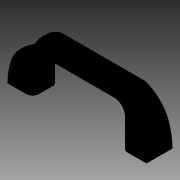
# Autodesk Inventor part: 2062
Saved by Autodesk Inventor 2014 SP2 (Build 180246200, 246)
## iProperties
Created: 2018-07-23
Part Number: 2062
Material: Generic
Catalog Web Link: www.cadenas.de
Description: 2060, 2061, 2062, 2880, 2881, 2882-Plastic Door Handles
Vendor: 8020
Document SubType Name: Modeling
Designer: psadmin
Manufacturer: 8020
Mass: 22.5234 g
Surface Area: 109.46 cm^2
Volume: 22.5234 cm^3
Density: 1 g/cm^3
Appearance: PSOLRGB-0-0-0
Category: PARTsolutions
Company: 8020
Title: 2062
Author: Cadenas PARTsolutions
Comments: Plastic Door Handles
PSOL_IDENT_0: {$CADENAS_DATA\23d-libs\8020\inch\panels_and_doors\2060.prj},182 {VTYP=3D},{NB=2062},{LINA=2062},{NN=
PSOL_IDENT_1: 2060, 2061, 2062, 2880, 2881, 2882},{DATE=16.03.2018 08:23:48},{GEOMDATE=03.01.2012 00:00:00},{VERSI
PSOL_IDENT_2: ON=},{LINEID=330},{WBVAR=COLOR},{WBNUMERIC=}  {NB=2062},{LINA=2062},{KT=DUMMY},{PN=2062},{SIZE=Small
PSOL_IDENT_3: },{MAT=High Strength Polycarbonate},{COLOR=Black},{A=4.409},{B=2.815},{C=1.417},{D=0.827},{E=3.681},
PSOL_IDENT_4: {F=1/4-20 SHCS (2)},{W=.055},{CC=6-10, 6-25},{COL=0.00,0.00,0.00,0.00}
NN: 2060, 2061, 2062, 2880, 2881, 2882
NT: Plastic Door Handles
NB: 2062
NBSYN: $PN.
LINA: 2062
PN: 2062
SIZE: Small
MAT: High Strength Polycarbonate
COLOR: Black
A: 4.409
B: 2.815
C: 1.417
D: 0.827
E: 3.681
F: 1/4-20 SHCS (2)
W: .055
CC: 6-10, 6-25
SUPPLIER: 8020
ARTICLENO: 2062
BOMINFO: 2062
CREATOR: CADENAS GmbH
Autodesk Inventor part; units mm, degrees
ref_plane "YZ Plane" through (0, 0, 0) normal (1, 0, 0) x (0, 1, 0)
ref_plane "XZ Plane" through (0, 0, 0) normal (0, 1, 0) x (-1, 0, 0)
ref_plane "XY Plane" through (0, 0, 0) normal (0, 0, 1) x (1, 0, 0)
sketch "Sketch_19" plane through (0, 0, 0) normal (0, 1, 0) x (-1, 0, 0)
  line L0 (20.2438, -10.5029) -> (20.2438, 10.5029)
  line L1 (20.2438, 10.5029) -> (5, 10.5029)
  arc A0 (5, 10.5029) -> (0, 5.5029) centre (5, 5.5029) ccw
  line L2 (0, 5.5029) -> (0, -5.5029)
  arc A1 (0, -5.5029) -> (5, -10.5029) centre (5, -5.5029) ccw
  line L3 (5, -10.5029) -> (20.2438, -10.5029)
  constraints: 8 end point, 4 point on circle, 2 centre point
extrude "Extrusion1" add sketch "Sketch_19" along normal blind 22.9918
sketch "Sketch_20" plane through (0, 22.9918, 0) normal (0, 1, 0) x (1, 0, 0)
  line L0 (7, 5.5029) -> (7, -5.5029)
  line L1 (-20.2438, 10.5029) -> (-20.2438, -10.5029)
  line L2 (-20.2438, -10.5029) -> (-5, -10.5029)
  arc A0 (-5, -10.5029) -> (0, -5.5029) centre (-5, -5.5029) ccw
  line L3 (0, -5.5029) -> (0, 5.5029)
  arc A1 (0, 5.5029) -> (-5, 10.5029) centre (-5, 5.5029) ccw
  line L4 (-5, 10.5029) -> (-20.2438, 10.5029)
  constraints: 10 end point, 4 point on circle, 2 centre point
revolve "Revolution1" add sketch "Sketch_20" angle 90 about axis through (7, 22.9918, -5.5029) along (0, 0, -1)
sketch "Sketch_21" plane through (7, 0, 0) normal (1, 0, 0) x (0, 0, -1)
  arc A0 (-10.5029, 34.9918) -> (-5.5029, 29.9918) centre (-5.5029, 34.9918) ccw
  line L0 (-5.5029, 29.9918) -> (5.5029, 29.9918)
  arc A1 (5.5029, 29.9918) -> (10.5029, 34.9918) centre (5.5029, 34.9918) ccw
  line L1 (10.5029, 34.9918) -> (10.5029, 50.2356)
  line L2 (10.5029, 50.2356) -> (-10.5029, 50.2356)
  line L3 (-10.5029, 50.2356) -> (-10.5029, 34.9918)
  constraints: 8 end point, 4 point on circle, 2 centre point
extrude "Extrusion2" add sketch "Sketch_21" along normal blind 57.501
sketch "Sketch_22" plane through (64.501, 0, 0) normal (1, 0, 0) x (0, 0, -1)
  line L0 (5.5029, 22.9918) -> (-5.5029, 22.9918)
  arc A0 (-10.5029, 34.9918) -> (-5.5029, 29.9918) centre (-5.5029, 34.9918) ccw
  line L1 (-5.5029, 29.9918) -> (5.5029, 29.9918)
  arc A1 (5.5029, 29.9918) -> (10.5029, 34.9918) centre (5.5029, 34.9918) ccw
  line L2 (10.5029, 34.9918) -> (10.5029, 50.2356)
  line L3 (10.5029, 50.2356) -> (-10.5029, 50.2356)
  line L4 (-10.5029, 50.2356) -> (-10.5029, 34.9918)
  constraints: 10 end point, 4 point on circle, 2 centre point
revolve "Revolution2" add sketch "Sketch_22" angle 90 about axis through (64.501, 22.9918, -5.5029) along (0, 0, -1)
sketch "Sketch_23" plane through (0, 0, 0) normal (0, 1, 0) x (-1, 0, 0)
  arc A0 (-71.501, 5.5029) -> (-76.501, 10.5029) centre (-76.501, 5.5029) ccw
  line L0 (-76.501, 10.5029) -> (-91.7448, 10.5029)
  line L1 (-91.7448, 10.5029) -> (-91.7448, -10.5029)
  line L2 (-91.7448, -10.5029) -> (-76.501, -10.5029)
  arc A1 (-76.501, -10.5029) -> (-71.501, -5.5029) centre (-76.501, -5.5029) ccw
  line L3 (-71.501, -5.5029) -> (-71.501, 5.5029)
  constraints: 8 end point, 4 point on circle, 2 centre point
extrude "Extrusion3" add sketch "Sketch_23" along normal blind 22.9918
sketch "Sketch_24" plane through (0, 0, 0) normal (0, 0, 1) x (1, 0, 0)
  line L0 (-32.9438, 71.9836) -> (-32.9438, 0)
  line L1 (-32.9438, 0) -> (-20.2438, 0)
  arc A0 (-18.4912, 13.0048) -> (-20.2438, 0) centre (34.459, -0.7516) ccw
  arc A1 (2.0066, 35.9918) -> (-18.4912, 13.0048) centre (10.8872, 7.4403) ccw
  line L2 (2.0066, 35.9918) -> (69.4944, 35.9918)
  arc A2 (89.9922, 13.0048) -> (69.4944, 35.9918) centre (60.6138, 7.4403) ccw
  arc A3 (91.7448, 0) -> (89.9922, 13.0048) centre (37.042, -0.7516) ccw
  line L3 (91.7448, 0) -> (104.4448, 0)
  line L4 (104.4448, 0) -> (104.4448, 71.9836)
  line L5 (104.4448, 71.9836) -> (-32.9438, 71.9836)
  constraints: 12 end point, 8 point on circle, 4 centre point
extrude "Extrusion4" cut sketch "Sketch_24" along normal mid plane 42.0116
sketch "Sketch_25" plane through (0, 0, 0) normal (0, 0, 1) x (1, 0, 0)
  line L0 (82.4992, 0) -> (82.4992, 35.9918)
  line L1 (82.4992, 35.9918) -> (87.7492, 35.9918)
  line L2 (87.7492, 35.9918) -> (87.7492, 6)
  line L3 (87.7492, 6) -> (85.7492, 6)
  line L4 (85.7492, 6) -> (85.7492, 0)
  line L5 (85.7492, 0) -> (82.4992, 0)
  line L6 (82.4992, 0) -> (82.4992, 35.9918)
  constraints: 14 end point
revolve "Revolution3" cut sketch "Sketch_25" angle 360 about axis through (82.4992, 0, 0) along (0, -1, 0)
sketch "Sketch_26" plane through (0, 0, 0) normal (0, 0, 1) x (1, 0, 0)
  line L0 (-10.9982, 0) -> (-10.9982, 35.9918)
  line L1 (-10.9982, 35.9918) -> (-5.7482, 35.9918)
  line L2 (-5.7482, 35.9918) -> (-5.7482, 6)
  line L3 (-5.7482, 6) -> (-7.7482, 6)
  line L4 (-7.7482, 6) -> (-7.7482, 0)
  line L5 (-7.7482, 0) -> (-10.9982, 0)
  line L6 (-10.9982, 0) -> (-10.9982, 35.9918)
  constraints: 14 end point
revolve "Revolution4" cut sketch "Sketch_26" angle 360 about axis through (-10.9982, 0, 0) along (0, -1, 0)
sketch "Sketch_27" plane through (0, 35.9918, 0) normal (0, 1, 0) x (1, 0, 0)
  line L0 (-32.9438, 23.2029) -> (-32.9438, -7.5)
  line L1 (-32.9438, -7.5) -> (-5, -7.5)
  arc A0 (-5, -7.5) -> (-3, -5.5) centre (-5, -5.5) ccw
  line L2 (-3, -5.5) -> (-3, 5.5)
  arc A1 (-3, 5.5) -> (-5, 7.5) centre (-5, 5.5) ccw
  line L3 (-5, 7.5) -> (-20.2438, 7.5)
  line L4 (-20.2438, 7.5) -> (-20.2438, 10.5029)
  line L5 (-20.2438, 10.5029) -> (91.7448, 10.5029)
  line L6 (91.7448, 10.5029) -> (91.7448, 7.5)
  line L7 (91.7448, 7.5) -> (76.501, 7.5)
  arc A2 (76.501, 7.5) -> (74.501, 5.5) centre (76.501, 5.5) ccw
  line L8 (74.501, 5.5) -> (74.501, -5.5)
  arc A3 (74.501, -5.5) -> (76.501, -7.5) centre (76.501, -5.5) ccw
  line L9 (76.501, -7.5) -> (104.4448, -7.5)
  line L10 (104.4448, -7.5) -> (104.4448, 23.2029)
  line L11 (104.4448, 23.2029) -> (-32.9438, 23.2029)
  constraints: 24 end point, 8 point on circle, 4 centre point
extrude "Extrusion5" cut sketch "Sketch_27" against normal blind 23
body "Solid1"
